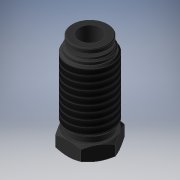
# Autodesk Inventor part: FVPA106J
Saved by Autodesk Inventor 2019 (Build 230136000, 136)
## iProperties
Created: 2023-10-05
Part Number: FVPA106J
Material: Generic
Catalog Web Link: www.cadenas.de
Description: Holder-
Vendor: PISCO_JP
Document SubType Name: Modeling
Designer: psAdmin
Manufacturer: PISCO_JP
Mass: 2.40056 g
Surface Area: 15.6611 cm^2
Volume: 2.40056 cm^3
Density: 1 g/cm^3
Appearance: PSOLRGB-175-175-175
Category: PARTsolutions
Company: PISCO_JP
Title: FVPA106J
Author: Cadenas PARTsolutions
PSOL_IDENT_0: {$CADENAS_DATA/23d-libs/pisco_jp/vacuum_pad_series_r2/holder_joint/parts/holder.prj},158 {VTYP=3D},{
PSOL_IDENT_1: NB=FVPA106J},{LINA=FVPA106J},{NN=Holder},{DATE=27.10.2022 04:02:53},{GEOMDATE=19.01.2021 07:54:00},{
PSOL_IDENT_2: VERSION=},{LINEID=2950},{WBVAR=},{WBNUMERIC=}  {NB=FVPA106J},{LINA=FVPA106J},{KT=DUMMY},{PARTNR=FVPA
PSOL_IDENT_3: 106J},{REF=VPA-M4-6J},{VER=13}
NB: FVPA106J
NN: Holder
NBSYN: $PARTNR.
LINA: FVPA106J
CATALOG: NIHON PISCO CO., LTD
PARTNR: FVPA106J
REF: VPA-M4-6J
VER: 13
SUPPLIER: PISCO_JP
ARTICLENO: FVPA106J
BOMINFO: FVPA106J
CREATOR: CADENAS GmbH
Autodesk Inventor part; units mm, degrees
sketch "Sketch_1" plane through (0, 0, 0) normal (0, 0, 1) x (1, 0, 0)
  line L0 (0, 0) -> (0, 5.5)
  line L1 (0, 5.5) -> (5.25, 5.5)
  line L2 (5.25, 5.5) -> (5.25, 4)
  line L3 (5.25, 4) -> (5.9, 4)
  line L4 (5.9, 4) -> (7.5, 3.0762)
  line L5 (7.5, 3.0762) -> (7.5, 0.9238)
  line L6 (7.5, 0.9238) -> (5.9, 0)
  line L7 (5.9, 0) -> (0, 0)
  line L8 (0, 0) -> (0, 5.5)
  constraints: 18 end point
revolve "Revolution1" add sketch "Sketch_1" angle 360 about axis through (0, 0, 0) along (0, -1, 0)
sketch "Sketch_2" plane through (0, 0, 0) normal (0, 1, 0) x (-1, 0, 0)
  line L0 (17.2177, 15.6183) -> (-16.6532, 15.6183)
  line L1 (-16.6532, 15.6183) -> (-16.6532, -14.1129)
  line L2 (-16.6532, -14.1129) -> (17.2177, -14.1129)
  line L3 (17.2177, -14.1129) -> (17.2177, 15.6183)
  line L4 (6.9282, 0) -> (3.4641, 6)
  line L5 (3.4641, 6) -> (-3.4641, 6)
  line L6 (-3.4641, 6) -> (-6.9282, 0)
  line L7 (-6.9282, 0) -> (-3.4641, -6)
  line L8 (-3.4641, -6) -> (3.4641, -6)
  line L9 (3.4641, -6) -> (6.9282, 0)
  constraints: 20 end point
extrude "Extrusion1" cut sketch "Sketch_2" along normal blind 4
sketch "Sketch_3" plane through (0, 0, 0) normal (0, 0, 1) x (1, 0, 0)
  line L0 (0, 5.5) -> (0, 26.1)
  line L1 (0, 26.1) -> (4.7, 26.1)
  arc A0 (4.9, 25.9) -> (4.7, 26.1) centre (4.7, 25.9) ccw
  line L2 (4.9, 25.9) -> (4.9, 24.9)
  line L3 (4.9, 24.9) -> (3.5, 24.9)
  line L4 (3.5, 24.9) -> (3.5, 24)
  line L5 (3.5, 24) -> (4.8, 24)
  line L6 (4.8, 24) -> (4.934, 23.5)
  line L7 (4.934, 23.5) -> (5.4, 23.2309)
  line L8 (5.4, 23.2309) -> (5.4, 22.5)
  line L9 (5.4, 22.5) -> (5.5, 22.5)
  line L10 (5.5, 22.5) -> (6, 22)
  line L11 (6, 22) -> (6, 6.25)
  line L12 (6, 6.25) -> (5.25, 5.5)
  line L13 (5.25, 5.5) -> (0, 5.5)
  line L14 (0, 5.5) -> (0, 26.1)
  constraints: 30 end point, 2 point on circle, 1 centre point
revolve "Revolution2" add sketch "Sketch_3" angle 360 about axis through (0, 5.5, 0) along (0, -1, 0)
thread "Thread1" size "M12x1.75" class "6g" standard "ISO Metric profile" full length
sketch "Sketch_4" plane through (0, 0, 0) normal (0, 0, 1) x (1, 0, 0)
  line L0 (0, 14.4) -> (0, 26.1)
  line L1 (0, 26.1) -> (3, 26.1)
  line L2 (3, 26.1) -> (3, 14.4)
  line L3 (3, 14.4) -> (0, 14.4)
  line L4 (0, 14.4) -> (0, 26.1)
  constraints: 10 end point
revolve "Revolution3" cut sketch "Sketch_4" angle 360 about axis through (0, 14.4, 0) along (0, -1, 0)
sketch "Sketch_5" plane through (0, 0, 0) normal (0, 0, 1) x (1, 0, 0)
  line L0 (0, 0) -> (0, 6.25)
  line L1 (0, 6.25) -> (1.621, 6.25)
  line L2 (1.621, 6.25) -> (1.621, 0)
  line L3 (1.621, 0) -> (0, 0)
  line L4 (0, 0) -> (0, 6.25)
  constraints: 10 end point
revolve "Revolution4" cut sketch "Sketch_5" angle 360 about axis through (0, 0, 0) along (0, -1, 0)
thread "Thread2" size "M4x0.7" class "6H" standard "ISO Metric profile" full length
ref_plane "IP_DUMMY_XY" through (0, 0, 0) normal (0, 1, 0) x (1, 0, 0)
ref_plane "IP_DUMMY_YZ" through (0, 0, 0) normal (1, 0, 0) x (0, 0, -1)
ref_plane "IP_DUMMY_ZX" through (0, 0, 0) normal (0, 0, -1) x (0, 1, 0)
ref_plane "IP_NUT1_XY" through (0, 11, 0) normal (0, 1, 0) x (1, 0, 0)
ref_plane "IP_NUT1_YZ" through (0, 11, 0) normal (1, 0, 0) x (0, 0, -1)
ref_plane "IP_NUT1_ZX" through (0, 11, 0) normal (0, 0, -1) x (0, 1, 0)
ref_plane "IP_NUT2_XY" through (0, 17, 0) normal (0, 1, 0) x (1, 0, 0)
ref_plane "IP_NUT2_YZ" through (0, 17, 0) normal (1, 0, 0) x (0, 0, -1)
ref_plane "IP_NUT2_ZX" through (0, 17, 0) normal (0, 0, -1) x (0, 1, 0)
body "Solid1"
